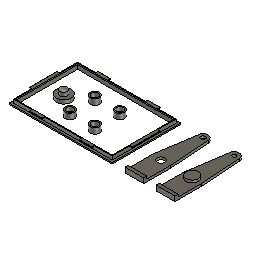
LCD_Bezel (Autodesk Fusion 360 design; units mm, degrees)
Autodesk Fusion 360 part; units mm, degrees
sketch "bezel face" plane through (0, 0, 0) normal (0, 0, 1) x (1, 0, 0) in component " clip in frame"
  line L0 (39.9, -26) -> (-39.9, -26)
  line L1 (-39.9, -26) -> (-39.9, 26)
  line L2 (-39.9, 26) -> (39.9, 26)
  line L3 (39.9, 26) -> (39.9, -26)
  line L4 (39.9, -26) -> (-39.9, 26) construction
  line L5 (-39.9, -26) -> (39.9, 26) construction
  line L6 (-38.4, -24.5) -> (-38.4, 24.5)
  line L7 (-38.4, 24.5) -> (38.4, 24.5)
  line L8 (38.4, 24.5) -> (38.4, -24.5)
  line L9 (38.4, -24.5) -> (-38.4, -24.5)
  line L10 (-41.4, -27.5) -> (-41.4, 27.5)
  line L11 (-41.4, 27.5) -> (41.4, 27.5)
  line L12 (41.4, 27.5) -> (41.4, -27.5)
  line L13 (41.4, -27.5) -> (-41.4, -27.5)
  point P0 (-39.9, -26)
  dimension "d1" = 79.8
  dimension "d2" = 52
  dimension "d55" = 1.5
  dimension "d56" = -1.5
  constraint parallel L0 L2
  constraint parallel L1 L3
  constraint horizontal L0
  constraint coincident P0 L0.end
  measures "d1" distance of L1.end L2.end
  measures "d2" distance of P0 L1.end
extrude "Extrude22" add sketch "bezel face" along normal blind 3.75 contours L0 L1 L2 L3 makes body 1 in component " clip in frame"
extrude "Extrude23" add sketch "bezel face" along normal blind 2 contours L10 L11 L12 L13 bodies 1 in component " clip in frame"
chamfer "Chamfer6" distance 1 angle 45 8 edges at (0, -24.5, 0) (0, -27.5, 0) (-41.4, 0, 0) (-38.4, 0, 0) (0, 24.5, 0) (0, 27.5, 0) (38.4, 0, 0) (41.4, 0, 0) on bodies 1 in component " clip in frame"
sketch "tab face" plane through (0, 0, 3.75) normal (0, 0, 1) x (-1, 0, 0) in component " clip in frame"
  line L0 (-38.4, -24.5) -> (-38.4, 24.5)
  line L1 (-38.4, 24.5) -> (38.4, 24.5)
  line L2 (38.4, 24.5) -> (38.4, -24.5)
  line L3 (38.4, -24.5) -> (-38.4, -24.5)
  line L4 (-39.9, -26) -> (39.9, -26)
  line L5 (39.9, -26) -> (39.9, 26)
  line L6 (39.9, 26) -> (-39.9, 26)
  line L7 (-39.9, 26) -> (-39.9, -26)
  line L8 (38.4, 24.5) -> (38.4, -24.5)
  line L9 (41.4, -27.5) -> (41.4, 27.5)
  line L10 (38.4, -24.5) -> (-38.4, -24.5)
  line L11 (-41.4, -27.5) -> (41.4, -27.5)
  line L12 (-38.4, 24.5) -> (38.4, 24.5)
  line L13 (41.4, 27.5) -> (-41.4, 27.5)
  line L14 (-38.4, -24.5) -> (-38.4, 24.5)
  line L15 (-41.4, 27.5) -> (-41.4, -27.5)
  line L16 (24.9, -11) -> (54.9, -11)
  line L17 (54.9, -11) -> (54.9, -41)
  line L18 (54.9, -41) -> (24.9, -41)
  line L19 (24.9, -41) -> (24.9, -11)
  line L20 (24.9, -11) -> (54.9, -41) construction
  line L21 (54.9, -11) -> (24.9, -41) construction
  point P0 (-39.9, -26)
  point P1 (-39.9, 26)
  point P2 (39.9, 26)
  point P3 (39.9, -26)
  dimension "d162" = 30
  dimension "d163" = 30
  constraint perpendicular L16 L17
  constraint parallel L16 L18
  constraint parallel L17 L19
  constraint horizontal L16
  constraint coincident L20 P3
  constraint coincident L21 P3
  constraint coincident P3 L4.end
  measures "d162" distance of L16.end L17.end
  measures "d163" distance of L17.end L18.end
extrude "Extrude24" add sketch "tab face" along normal blind 1 contours L0 L1 L2 L3 L4 L5 L6 L7 L8 L10 L12 L14 L16 L19 | L2 L3 L4 L5 L8 L10 L16 L19 | L4 L5 L6 L7 L9 L11 L13 L15 L16 L19 | L4 L5 L9 L11 L16 L19 bodies 1 in component " clip in frame"
chamfer "Chamfer7" distance 0.5 distance2 1 4 edges at (0, -27.5, 3.75) (41.4, 0, 3.75) (0, 27.5, 3.75) (-41.4, 0, 3.75) measured on face at (-13.8, -27.5, 4.0833) measured on face at (41.4, -9.1667, 4.0833) measured on face at (13.8, 27.5, 4.0833) measured on face at (-41.4, 9.1667, 4.0833) on bodies 1 in component " clip in frame"
extrude "Extrude30" cut sketch "tab face" along normal blind 1 contours L2 L3 L8 L10 L16 L19 | L2 L3 L4 L5 L8 L10 L16 L19 | L4 L5 L9 L11 L16 L19 | L9 L11 L16 L17 L18 L19 bodies 1 in component " clip in frame"
pattern_linear "R-Pattern8" count 3 spacing 39.9 along (1, 0, 0) count 2 spacing 52 along (0, -1, 0) of "Extrude30" in component " clip in frame"
move_face "OffsetFaces3" offset -0.3 4 faces at (39.9, 3.6667, 2.5833) (8.3, -26, 2.5833) (-39.9, -3.6667, 2.5833) (-8.3, 26, 2.5833) on bodies 1 in component " clip in frame"
extrude "Extrude33" add 6 faces at (-39.2, 20.4, 3.75) (5, 25.3, 3.75) (-39.2, -20.4, 3.75) (5, -25.3, 3.75) (39.2, 20.4, 3.75) (39.2, -20.4, 3.75) along direction (0, 0, 1) up to surface end surface through (0, 0, 4.75) normal (0, 0, 1) offset 0 on bodies 1 bodies 1 in component " clip in frame"
fillet "Fillet3" radius 0.5 4 edges at (-38.4, 0, 4.75) (0, 24.5, 4.75) (0, -24.5, 4.75) (38.4, 0, 4.75) on bodies 1 in component " clip in frame"
sketch "spacer" plane through (0, 0, 0) normal (0, 0, 1) x (1, 0, 0) in component "tab spacer"
  circle A0 centre (-10, 10) radius 1.625
  circle A1 centre (-10, 10) radius 2.75
  circle A2 centre (-10, 10) radius 3.75
  dimension "d43" = 3.25
  dimension "d44" = 5.5
  dimension "d45" = 7.5
  constraint concentric A0 A1
  constraint concentric A0 A2
  measures "d43" diameter of A0
  measures "d44" diameter of A1
  measures "d45" diameter of A2
extrude "Extrude1" add sketch "spacer" along normal blind 1 separate body contours A1 makes body 2 in component "tab spacer"
extrude "Extrude2" add sketch "spacer" along normal blind 4.5 contours A2 bodies 2 in component "tab spacer"
pattern_linear "ﬁ15" [suppressed]
sketch "button profile" plane through (0, 0, 0) normal (0, 1, 0) x (1, 0, 0) in component "button"
  arc A0 (0, -7) -> (3, -6) centre (0.25, -2.75) ccw
  line L0 (3, -6) -> (3, -3)
  line L1 (0, -7) -> (0, -3.0001)
  line L2 (3, -3.0001) -> (3, -3)
  line L3 (0, -3) -> (0, -3.0001)
  line L4 (1.75, -0.0001) -> (1.75, -2.5)
  line L5 (1.75, -2.5) -> (0, -2.5)
  line L6 (0, -3) -> (0, -2.5)
  line L7 (3, -3.0001) -> (6, -3.0001)
  line L8 (6, -3.0001) -> (6, -0.0001)
  line L9 (6, -0.0001) -> (1.75, -0.0001)
  dimension "d49_1" = 1.75
  dimension "d50_1" = 3
  dimension "d51_1" = 2.5
  dimension "d52_1" = 3.9999
  dimension "d53_1" = 3
  dimension "d54" = 3
  dimension "d55_1" = 4.25
  dimension "d56_1" = 3
  dimension "d57" = 0.5
  constraint vertical L2
  constraint vertical L3
  constraint vertical L4
  constraint horizontal L5
  constraint perpendicular L5 L6
  constraint perpendicular L0 L7
  constraint perpendicular L5 L8
  constraint perpendicular L4 L9
  measures "d49_1" distance of origin L4.start
  measures "d50_1" distance of L2.start L7.end
  measures "d51_1" distance of origin L5.end
  measures "d52_1" distance of A0.start L1.end
  measures "d53_1" distance of A0.end L0.end
  measures "d54" distance of L7.end L8.end
  measures "d55_1" distance of L4.start L8.end
  measures "d56_1" distance of L0 L1
  measures "d57" distance of L3.start L5.end
revolve "Revolve3" [suppressed] in component "button"
revolve "Revolve4" add sketch "button profile" angle 360 about axis through (0, 0, 1.75) along (0, 0, 1) separate body makes body 3 in component "button"
sketch "jig" plane through (0, 0, 0) normal (0, 0, 1) x (1, 0, 0) in component "testing jig"
  line L0 (0, 0) -> (21.5431, 0)
  line L1 (21.9831, 15) -> (0, 15)
  line L2 (0, 15) -> (0, 0)
  line L3 (0, 0) -> (2.5, 0)
  line L4 (2.5, 0) -> (2.5, 15.01)
  line L5 (2.5, 15.01) -> (0, 15.01)
  line L6 (0, 15.01) -> (0, 0)
  line L7 (2.5, 7.505) -> (21.4, 7.505) construction
  circle A0 centre (21.4, 7.505) radius 5
  line L8 (21.4, 7.505) -> (53.8, 7.505) construction
  line L9 (53.8, 7.505) -> (53.8, 6.166) construction
  circle A1 centre (53.8, 6.166) radius 1.75
  line L10 (21.9831, 15) -> (54.3955, 10.1197)
  line L11 (21.5431, 0) -> (54.0661, 2.1766)
  arc A2 (54.0661, 2.1766) -> (54.3955, 10.1197) centre (53.8, 6.166) ccw
  circle A3 centre (21.4, 7.505) radius 3
  circle A4 centre (53.5, 5.5) radius 0.1394
  dimension "d2_1" = 15
  dimension "d3" = 2.5
  dimension "d4" = 18.9
  dimension "d5" = 10
  dimension "d6" = 32.4
  dimension "d7" = 1.339
  dimension "d8" = 3.5
  dimension "d21" = 6
  constraint horizontal L0
  constraint horizontal L1
  constraint vertical L2
  constraint coincident L0.start L2.end
  constraint horizontal L3
  constraint vertical L4
  constraint horizontal L5
  constraint vertical L6
  constraint midpoint L4 L7.start
  constraint perpendicular L4 L7
  constraint coincident L7.end A0.centre
  constraint parallel L7 L8
  constraint perpendicular L8 L9
  constraint coincident L9.end A1.centre
  constraint concentric A0 A3
  measures "d2_1" distance of L0.start L1.end
  measures "d3" distance of L0.start L3.end
  measures "d4" distance of L7.start L7.end
  measures "d5" diameter of A0
  measures "d6" distance of L7.end L8.end
  measures "d7" distance of L8.end L9.end
  measures "d8" diameter of A1
  measures "d21" diameter of A3
extrude "Extrude1'" add sketch "jig" along normal blind 2 separate body contours L0 L1 L2 L3 L4 L6 makes body 4 in component "testing jig"
extrude "Extrude2'" add sketch "jig" against normal blind 2 contours L0 L1 L2 L3 L4 L6 | L0 L1 L4 L10 L11 A2 | A0 bodies 4 in component "testing jig"
sketch "text" plane through (0, 0, -2) normal (0, 0, -1) x (1, 0, 0) in component "testing jig"
  circle A0 centre (53.8, -6.166) radius 1.75
  line L0 (0, -15) -> (21.9831, -15)
  line L1 (21.9831, -15) -> (54.3955, -10.1197)
  arc A1 (54.3955, -10.1197) -> (54.0661, -2.1766) centre (53.8, -6.166) ccw
  line L2 (54.0661, -2.1766) -> (21.5431, 0)
  line L3 (21.5431, 0) -> (0, 0)
  line L4 (0, 0) -> (0, -15)
  line L5 (6.5378, -10.9721) -> (5.4173, -9.0313)
  line L6 (7.6583, -9.0313) -> (6.5378, -10.9721)
  line L7 (6.25, -9.0313) -> (6.25, -4.3533)
  line L8 (6.25, -4.3533) -> (6.75, -4.3533)
  line L9 (6.75, -4.3533) -> (6.75, -9.0313)
  line L10 (5.4173, -9.0313) -> (6.25, -9.0313)
  line L11 (6.75, -9.0313) -> (7.6583, -9.0313)
  circle A2 centre (21.4, -7.505) radius 3
  point P0 (6.5, -7)
  dimension "d17" = 0.5
  constraint equal L5 L6
  constraint parallel L7 L9
  constraint collinear L10 L11
  measures "d17" distance of L7.end L8.end
extrude "Extrude4" cut sketch "text" against normal blind 0.5 contours L5 L6 L7 L8 L9 L10 L11 bodies 4 in component "testing jig"
move_face "OffsetFaces2" offset -0.1 2 faces at (24.3963, 7.3555, -1.3333) (53.2426, 4.5071, -1.3333) on bodies 4 in component "testing jig"
sketch "jig (2)" plane through (0, 0, 0) normal (0, 0, 1) x (1, 0, 0) in component "marking jig"
  line L0 (0, 0) -> (21.5682, 0)
  line L1 (21.9273, 15) -> (0, 15)
  line L2 (0, 15) -> (0, 0)
  line L3 (0, 0) -> (2.5, 0)
  line L4 (2.5, 0) -> (2.5, 15)
  line L5 (2.5, 15) -> (0, 15)
  line L6 (0, 15) -> (0, 0)
  line L7 (2.5, 7.5) -> (21.4, 7.5) construction
  circle A0 centre (21.4, 7.5) radius 4.995
  line L8 (21.4, 7.5) -> (53.8, 7.5) construction
  line L9 (53.8, 7.5) -> (53.8, 6.161) construction
  circle A1 centre (53.8, 6.161) radius 1.5
  line L10 (21.8001, 2.521) -> (53.8999, 4.6643) construction
  line L11 (22.1429, 12.4394) -> (54.0231, 7.6443) construction
  line L12 (21.9273, 15) -> (54.395, 10.1165)
  line L13 (21.5682, 0) -> (54.0665, 2.1699)
  arc A2 (54.0665, 2.1699) -> (54.395, 10.1165) centre (53.8, 6.161) ccw
  dimension "d2_2" = 15
  dimension "d3_1" = 2.5
  dimension "d4_1" = 18.9
  dimension "d5_1" = 9.99
  dimension "d6_1" = 32.4
  dimension "d7_1" = 1.339
  dimension "d8_1" = 3
  constraint horizontal L0
  constraint horizontal L1
  constraint vertical L2
  constraint coincident L0.start L2.end
  constraint horizontal L3
  constraint vertical L4
  constraint horizontal L5
  constraint vertical L6
  constraint midpoint L4 L7.start
  constraint perpendicular L4 L7
  constraint coincident L7.end A0.centre
  constraint parallel L7 L8
  constraint perpendicular L8 L9
  constraint coincident L9.end A1.centre
  constraint coincident A0 L10.start
  constraint coincident A1 L10.end
  constraint tangent A1 L10
  constraint coincident A0 L11.start
  constraint coincident A1 L11.end
  constraint tangent A1 L11
  constraint tangent A0 L11
  constraint parallel L11 L12
  constraint parallel L10 L13
  measures "d2_2" distance of L0.start L1.end
  measures "d3_1" distance of L0.start L3.end
  measures "d4_1" distance of L7.start L7.end
  measures "d5_1" diameter of A0
  measures "d6_1" distance of L7.end L8.end
  measures "d7_1" distance of L8.end L9.end
  measures "d8_1" diameter of A1
extrude "Extrude1''" add sketch "jig (2)" along normal blind 2 separate body contours L0 L1 L2 L3 L4 L5 L6 | A0 makes body 5 at (0.8333, 10, 0) makes body 6 at (23.857, 6.5592, 0) in component "marking jig"
extrude "Extrude2''" add sketch "jig (2)" against normal blind 2 contours L0 L1 L2 L3 L4 L5 L6 | L0 L1 L4 L12 L13 A2 | A0 bodies 5 6 in component "marking jig"
sketch "text (2)" plane through (0, 0, -2) normal (0, 0, -1) x (1, 0, 0) in component "marking jig"
  circle A0 centre (53.8, -6.161) radius 1.5
  line L0 (0, -15) -> (21.9273, -15)
  line L1 (21.9273, -15) -> (54.395, -10.1165)
  arc A1 (54.395, -10.1165) -> (54.0665, -2.1699) centre (53.8, -6.161) ccw
  line L2 (54.0665, -2.1699) -> (21.5682, 0)
  line L3 (21.5682, 0) -> (0, 0)
  line L4 (0, 0) -> (0, -15)
  line L5 (22, -5) -> (10.0088, -5) construction
  line L6 (10.0088, -5) -> (10.0088, -11) construction
  line L7 (10.0088, -11) -> (22, -11) construction
  line L8 (22, -11) -> (22, -5) construction
  line L9 (6.5378, -10.9721) -> (5.4173, -9.0313)
  line L10 (7.6583, -9.0313) -> (6.5378, -10.9721)
  line L11 (6.25, -9.0313) -> (6.25, -4.3533)
  line L12 (6.25, -4.3533) -> (6.75, -4.3533)
  line L13 (6.75, -4.3533) -> (6.75, -9.0313)
  line L14 (5.4173, -9.0313) -> (6.25, -9.0313)
  line L15 (6.75, -9.0313) -> (7.6583, -9.0313)
  point P0 (6.5, -7)
  dimension "d17_1" = 0.5
  text T0 "TOP " font "Arial" height 6 bold align ink ink in box 0 x 0 at (22, -5) x (-1, 0) y (0, -1) spacing 1 kerned height is em
  constraint perpendicular L5 L6
  constraint parallel L5 L7
  constraint parallel L6 L8
  constraint equal L9 L10
  constraint parallel L11 L13
  constraint collinear L14 L15
  measures "d17_1" distance of L11.end L12.end
extrude "Extrude3" cut sketch "text (2)" against normal blind 0.5 text T0 bodies 5 in component "marking jig"
extrude "Extrude4'" cut sketch "text (2)" against normal blind 0.5 contours L9 L10 L11 L12 L13 L14 L15 bodies 5 in component "marking jig"
move_face "OffsetFaces1" offset -0.1 1 faces at (26.3888, 7.251, 1.3333) on bodies 5 in component "marking jig"
component " clip in frame" placed x (1, 0, 0) y (0, 1, 0) z (0, 0, 1) at (0, 0, 0)
component "tab spacer" placed x (1, 0, 0) y (0, 1, 0) z (0, 0, 1) at (0, 0, 0)
component "tab spacer" placed x (1, 0, 0) y (0, 1, 0) z (0, 0, 1) at (20, 0, 0)
component "tab spacer" placed x (1, 0, 0) y (0, 1, 0) z (0, 0, 1) at (0, -20, 0)
component "tab spacer" placed x (1, 0, 0) y (0, 1, 0) z (0, 0, 1) at (20, -20, 0)
component "button" placed x (1, 0, 0) y (0, 1, 0) z (0, 0, 1) at (-25, 0, 0)
component "testing jig" placed x (0, 1, 0) y (-1, 0, 0) z (0, 0, 1) at (66.7857, -27.4723, 2)
component "marking jig" placed x (0, 1, 0) y (-1, 0, 0) z (0, 0, 1) at (91.7857, -27.4723, 2)
equation "d1 = openingWidth"
equation "d2 = openingHeight"
equation "openingWidth = 79.8 mm"
equation "openingHeight = 52 mm"
equation "panelThickness = 1.75 mm"
equation "d126 = panelThickness + bezelHeight"
equation "bezelHeight = 2 mm"
equation "d129 = bezelHeight"
equation "d132 = tabThickness"
equation "tabThickness = 1 mm"
equation "d164 = tabThickness"
equation "d168 = openingWidth"
equation "d169 = -openingHeight"
equation "postDiameter = 5.5 mm"
equation "d44 = postDiameter"
equation "d45 = postDiameter + 2 mm"
equation "d46 = tabThickness"
equation "d48 = tabThickness + 3.5 mm"
named bodies: "bezel", "spacer", "button", "jig"
